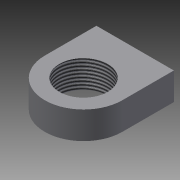
# Autodesk Inventor part: AcmeMountingFlange
Saved by Autodesk Inventor 2013 (Build 170138000, 138)
## iProperties
Created: 2012-12-09
Part Number: AcmeMountingFlange
Material: Generic
Document SubType Name: Modeling
Designer: Istvan
Density: 1 g/cm^3
Mass: 14.7064 g
Surface Area: 51.9439 cm^2
Volume: 14.7064 cm^3
Author: Istvan
Autodesk Inventor part; units mm, degrees
ref_plane "YZ Plane" through (0, 0, 0) normal (1, 0, 0) x (0, 1, 0)
ref_plane "XZ Plane" through (0, 0, 0) normal (0, 1, 0) x (-1, 0, 0)
ref_plane "XY Plane" through (0, 0, 0) normal (0, 0, 1) x (1, 0, 0)
sketch "Sketch1" plane through (0, 0, 0) normal (0, 1, 0) x (-1, 0, 0)
  circle A0 centre (0, 0) radius 11.9062
  arc A1 (19.05, 0) -> (-19.05, 0) centre (0, 0) ccw
  line L0 (19.05, 0) -> (19.05, -25.4)
  line L1 (19.05, -25.4) -> (-19.05, -25.4)
  line L2 (-19.05, -25.4) -> (-19.05, 0)
  dimension "d0" = 23.8125
  dimension "d2" = 38.1
  dimension "d16" = 25.4
  constraints: 6 end point, 2 centre point, 2 coincident, 2 horizontal alignment, 2 point on circle, 1 horizontal, 1 parallel, 1 vertical
  measures "d0" diameter of A0
  measures "d2" diameter of A1
  measures "d16" distance from line of L1 L2.end
extrude "Extrusion1" add sketch "Sketch1" along normal blind 13.462
thread "Thread1" size "15/16-16 UN" class "2B" standard "ANSI Unified Screw Threads" full length
body "Solid1"
